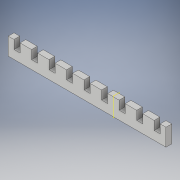
# Autodesk Inventor part: brace
Saved by Autodesk Inventor 2017 (Build 210142000, 142)
## iProperties
Created: 2017-05-09
Part Number: brace
Material: Generic
Document SubType Name: Modeling
Designer: s4461999
Density: 1 g/cm^3
Appearance: Default
Author: s4461999
Autodesk Inventor part; units mm, degrees
ref_plane "YZ Plane" through (0, 0, 0) normal (1, 0, 0) x (0, 1, 0)
ref_plane "XZ Plane" through (0, 0, 0) normal (0, 1, 0) x (-1, 0, 0)
ref_plane "XY Plane" through (0, 0, 0) normal (0, 0, 1) x (1, 0, 0)
sketch "Sketch1" plane through (0, 0, 0) normal (0, 0, 1) x (1, 0, 0)
  line L0 (0, 0) -> (0, 15)
  line L1 (0, 15) -> (5, 15)
  line L2 (5, 15) -> (5, 7.5)
  line L3 (5, 7.5) -> (10.2, 7.5)
  line L4 (10.2, 7.5) -> (10.2, 15)
  line L5 (10.2, 15) -> (15.2, 15)
  line L6 (15.2, 15) -> (15.2, 0)
  line L7 (15.2, 0) -> (0, 0)
  dimension "d0" = 15
  dimension "d1" = 5.2
  dimension "d2" = 5
  dimension "d3" = 5
  dimension "d4" = 7.5
  constraints: 16 end point, 6 perpendicular, 2 point on line, 1 vertical
  measures "d0" distance between parallel lines of L1 L7
  measures "d1" distance between parallel lines of L4 L2
  measures "d2" distance between parallel lines of L2 L0
  measures "d3" distance between parallel lines of L6 L4
  measures "d4" distance between parallel lines of L3 L1
extrude "Extrusion1" add sketch "Sketch1" along normal blind 5
mirror "Mirror1" about plane through (15.2, 0, 0) normal (1, 0, 0) of "Extrusion1"
mirror "Mirror2" about plane through (30.4, 15, 0) normal (1, 0, 0) of "Extrusion1", "Mirror1"
mirror "Mirror4" about plane through (0, 15, 0) normal (-1, 0, 0) of "Extrusion1"
mirror "Mirror5" about plane through (-15.2, 0, 0) normal (-1, 0, 0) of "Extrusion1", "Mirror4"
ref_plane "Work Plane3" through (45.6, 7.5, 0) normal (1, 0, 0) x (0, 0, -1)
mirror "Mirror7" about plane through (45.6, 7.5, 0) normal (1, 0, 0) of "Extrusion1", "Mirror1"
body "Solid1"
